Autodesk Inventor part; units mm, degrees
(part 2 of 2)
sketch "Sketch7" plane through (0, 0, 6) normal (0, 0, 1) x (1, 0, 0)
  line L0 (64, -15) -> (64, 15) projected
  line L1 (64, -15) -> (59, -15)
  line L2 (59, -15) -> (59, -10)
  line L3 (59, -10) -> (64, -10)
  line L4 (64, -10) -> (64, -15)
  line L5 (64, 15) -> (59, 15)
  line L6 (59, 15) -> (59, 10)
  line L7 (59, 10) -> (64, 10)
  line L8 (64, 10) -> (64, 15)
  line L9 (59, 10) -> (30, 10)
  line L10 (30, 10) -> (30, -10)
  line L11 (30, -10) -> (59, -10)
  line L12 (59, -10) -> (59, 10)
  line L13 (30, 10) -> (25, 10)
  line L14 (25, 10) -> (25, 15)
  line L15 (25, 15) -> (30, 15)
  line L16 (30, 15) -> (30, 10)
  line L17 (30, -10) -> (25, -10)
  line L18 (25, -10) -> (25, -15)
  line L19 (25, -15) -> (30, -15)
  line L20 (30, -15) -> (30, -10)
  line L21 (47, 2.5) -> (42, 2.5)
  line L22 (42, 2.5) -> (42, -2.5)
  line L23 (42, -2.5) -> (47, -2.5)
  line L24 (47, -2.5) -> (47, 2.5)
  line L25 (47, 2.5) -> (42, -2.5) construction
  line L26 (42, 2.5) -> (47, -2.5) construction
  line L27 (61.5, -10) -> (47, 0)
  line L28 (59, -12.5) -> (44.5, -2.5)
  line L29 (44.5, -2.5) -> (30, -12.5)
  line L30 (42, 0) -> (27.5, -10)
  line L31 (42, 0) -> (27.5, 10)
  line L32 (44.5, 2.5) -> (30, 12.5)
  line L33 (44.5, 2.5) -> (59, 12.5)
  line L34 (47, 0) -> (61.5, 10)
  point P0 (0, 0)
  point P1 (44.5, 0)
  point P2 (55.375, 10)
  point P3 (33.625, 10)
  point P4 (30, 8.2759)
  point P5 (30, -8.2759)
  point P6 (33.625, -10)
  point P7 (55.375, -10)
  point P8 (59, 8.2759)
  point P9 (59, -8.2759)
  dimension "d33" = 5
  dimension "d34" = 5
  dimension "d35" = 5
  dimension "d36" = 5
  dimension "d37" = 29
  dimension "d38" = 20
  dimension "d39" = 5
  dimension "d40" = 5
  dimension "d41" = 5
  dimension "d42" = 5
  dimension "d43" = 5
  dimension "d44" = 5
  constraints: 68 end point, 14 midpoint, 12 parallel, 6 horizontal, 6 perpendicular, 1 point on line
  measures "d33" distance of L2.end L3.end
  measures "d34" distance of L1.end L2.end
  measures "d35" distance of L7.end L6.end
  measures "d36" distance of L6.end L5.end
  measures "d37" distance of L11.end L10.end
  measures "d38" distance of L10.end L9.end
  measures "d39" distance of L14.end L15.end
  measures "d40" distance of L13.end L14.end
  measures "d41" distance of L19.end L18.end
  measures "d42" distance of L18.end L17.end
  measures "d43" distance of L23.end L22.end
  measures "d44" distance of L22.end L21.end
extrude "Extrusion7" cut sketch "Sketch7" against normal blind 6 contours L27 L34 L12 | L11 L29 L28 | L33 L32 L9 | L10 L31 L30
fillet "Fillet2" radius 1 12 edges at (59, -8.2759, 3) (44.5, -2.5, 3) (59, 8.2759, 3) (30, 8.2759, 3) (55.375, 10, 3) (55.375, -10, 3) (33.625, -10, 3) (30, -8.2759, 3) (42, 0, 3) (44.5, 2.5, 3) (47, 0, 3) (33.625, 10, 3)
sketch "Sketch8" plane through (0, 0, 6) normal (0, 0, 1) x (1, 0, 0)
  line L0 (30, -45) -> (30, -15) projected
  line L1 (30, -45) -> (0, -45)
  line L2 (0, -45) -> (0, 15.0455)
  line L3 (0, 15.0455) -> (30, 15.0455)
  line L4 (30, 15.0455) -> (30, -45)
  line L5 (30, -45) -> (25, -45)
  line L6 (25, -45) -> (25, 15.0455)
  line L7 (25, 15.0455) -> (30, 15.0455)
  line L8 (30, 15.0455) -> (30, -45)
  line L9 (25, -45) -> (0, -45)
  line L10 (0, -45) -> (0, -40)
  line L11 (0, -40) -> (25, -40)
  line L12 (25, -40) -> (25, -45)
  line L13 (25, 15.0455) -> (0, 15.0455)
  line L14 (0, 15.0455) -> (0, 10.0455)
  line L15 (0, 10.0455) -> (25, 10.0455)
  line L16 (25, 10.0455) -> (25, 15.0455)
  line L17 (0, -40) -> (2.5, -40)
  line L18 (2.5, -40) -> (2.5, 10.0455)
  line L19 (2.5, 10.0455) -> (0, 10.0455)
  line L20 (0, 10.0455) -> (0, -40)
  line L21 (2.5, -36.9397) -> (25, -36.9397)
  line L22 (25, -36.9397) -> (25, -31.9397)
  line L23 (25, -31.9397) -> (2.5, -31.9397)
  line L24 (2.5, -31.9397) -> (2.5, -36.9397)
  line L25 (25, -31.9397) -> (2.5, -31.9397)
  line L26 (2.5, -31.9397) -> (2.5, -26.9397)
  line L27 (2.5, -26.9397) -> (25, -26.9397)
  line L28 (25, -26.9397) -> (25, -31.9397)
  line L29 (2.5, -26.9397) -> (25, -26.9397)
  line L30 (25, -26.9397) -> (25, -21.9397)
  line L31 (25, -21.9397) -> (2.5, -21.9397)
  line L32 (2.5, -21.9397) -> (2.5, -26.9397)
  line L33 (25, -21.9397) -> (2.5, -21.9397)
  line L34 (2.5, -21.9397) -> (2.5, -16.9397)
  line L35 (2.5, -16.9397) -> (25, -16.9397)
  line L36 (25, -16.9397) -> (25, -21.9397)
  line L37 (25, 10.0455) -> (2.5, 10.0455)
  line L38 (2.5, 10.0455) -> (2.5, 5.0455)
  line L39 (2.5, 5.0455) -> (25, 5.0455)
  line L40 (25, 5.0455) -> (25, 10.0455)
  line L41 (2.5, 5.0455) -> (25, 5.0455)
  line L42 (25, 5.0455) -> (25, 0.0455)
  line L43 (25, 0.0455) -> (2.5, 0.0455)
  line L44 (2.5, 0.0455) -> (2.5, 5.0455)
  line L45 (25, 0.0455) -> (2.5, 0.0455)
  line L46 (2.5, 0.0455) -> (2.5, -4.9545)
  line L47 (2.5, -4.9545) -> (25, -4.9545)
  line L48 (25, -4.9545) -> (25, 0.0455)
  line L49 (2.5, -4.9545) -> (25, -4.9545)
  line L50 (25, -4.9545) -> (25, -9.9545)
  line L51 (25, -9.9545) -> (2.5, -9.9545)
  line L52 (2.5, -9.9545) -> (2.5, -4.9545)
  line L53 (25, -9.9545) -> (2.5, -9.9545)
  line L54 (2.5, -9.9545) -> (2.5, -16.9397)
  line L55 (2.5, -16.9397) -> (25, -16.9397)
  line L56 (25, -16.9397) -> (25, -9.9545)
  line L57 (16.2931, -16.9397) -> (16.2931, -4.9545)
  point P0 (0, 0)
  point P1 (16.2931, -9.9545)
  dimension "d48" = 5
  dimension "d49" = 5
  dimension "d50" = 5
  dimension "d51" = 2.5
  dimension "d52" = 5
  dimension "d53" = 5
  dimension "d54" = 5
  dimension "d55" = 5
  dimension "d56" = 5
  dimension "d57" = 5
  dimension "d58" = 5
  dimension "d59" = 5
  constraints: 114 end point, 28 parallel, 15 perpendicular, 15 point on line, 14 horizontal
  measures "d48" distance of L6.end L7.end
  measures "d49" distance of L9.end L10.end
  measures "d50" distance of L14.end L13.end
  measures "d51" distance of L19.end L18.end
  measures "d52" distance of L22.end L21.end
  measures "d53" distance of L25.end L26.end
  measures "d54" distance of L30.end L29.end
  measures "d55" distance of L33.end L34.end
  measures "d56" distance of L38.end L37.end
  measures "d57" distance of L41.end L42.end
  measures "d58" distance of L46.end L45.end
  measures "d59" distance of L49.end L50.end
extrude "Extrusion8" cut sketch "Sketch8" against normal blind 6 contours L21 L18 L23 L6 | L6 L39 L18 L15 | L27 L18 L31 L6 | L6 L47 L18 L43 | L35 L18 L51 L57
fillet "Fillet3" radius 2 20 edges at (25, -4.9545, 3) (25, 5.0455, 3) (16.2931, -16.9397, 3) (25, -26.9397, 3) (25, -21.9397, 3) (16.2931, -9.9545, 3) (25, 0.0455, 3) (25, 10.0455, 3) (2.5, 10.0455, 3) (2.5, 5.0455, 3) (2.5, 0.0455, 3) (2.5, -4.9545, 3) (2.5, -9.9545, 3) (2.5, -16.9397, 3) (2.5, -21.9397, 3) (2.5, -26.9397, 3) (2.5, -31.9397, 3) (2.5, -36.9397, 3) (25, -36.9397, 3) (25, -31.9397, 3)
mirror "Mirror2" about plane through (0, -15, 6) normal (-1, 0, 0) of "Fillet2", "Extrusion7", "Extrusion8", "Fillet3"
fillet "Fillet4" radius 2 6 edges at (-30, -15, 3) (-30, -45, 3) (30, -45, 3) (30, -15, 3) (-64, 0, 6) (64, 0, 6)
body "Solid1"
